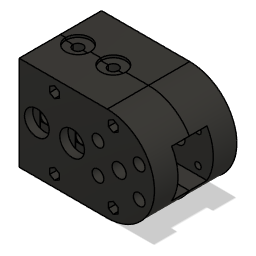
side brace lower mount v4 (Autodesk Fusion 360 design; units mm, degrees)
Autodesk Fusion 360 part; units mm, degrees
sketch "Sketch1" plane through (0, 0, 0) normal (0, 0, 1) x (1, 0, 0)
  line L0 (0, 20.1) -> (0, -20.1)
  line L1 (0, 20.1) -> (-60, 20.1)
  line L2 (-60, 20.1) -> (-60, 40.1)
  line L3 (-60, 40.1) -> (14.9, 40.1)
  circle A0 centre (25, 0) radius 6
  line L4 (0, -20.1) -> (-60, -20.1)
  line L5 (-60, -20.1) -> (-60, -40.1)
  line L6 (-60, -40.1) -> (14.9, -40.1)
  circle A1 centre (25, 0) radius 12.5
  line L7 (0, 0) -> (25, 0) construction
  line L8 (25, 0) -> (55, 0) construction
  arc A2 (14.9, -40.1) -> (14.9, 40.1) centre (14.9, 0) ccw
  dimension "d1" = 40.2
  dimension "d2" = 60
  dimension "d3" = 20
  dimension "d4" = 12
  dimension "d6" = 25
  dimension "d7" = 25
  dimension "d14" = 30
  constraint vertical L0
  constraint midpoint L7.start L0
  constraint perpendicular L0 L1
  constraint perpendicular L1 L2
  constraint perpendicular L2 L3
  constraint perpendicular L2 L4
  constraint perpendicular L1 L5
  constraint perpendicular L5 L6
  constraint equal L2 L5
  constraint collinear L2 L5
  constraint concentric A0 A1
  constraint coincident L7.start origin
  constraint coincident A0.centre A1.centre
  constraint horizontal L7
  constraint parallel L7 L8
  constraint coincident L7 A2.centre
  constraint tangent L3 A2
  constraint coincident L8.end A2
  measures "d1" distance of L0.start L0.end
  measures "d2" distance of L0.start L1.end
  measures "d3" distance of L1.end L2.end
  measures "d4" diameter of A0
  measures "d6" diameter of A1
  measures "d7" distance of L0 A0.centre
  measures "d14" distance of A0.centre L8.end
extrude "Extrude1" add sketch "Sketch1" along normal blind 20 contours L0 L1 L2 L3 L4 L5 L6 A2 | A1 makes body 1
sketch "Sketch3" plane through (0, 0, 0) normal (0, 0, -1) x (-1, 0, 0)
  circle A0 centre (-25, 0) radius 6
  line L0 (0, -20.1) -> (0, 20.1)
  line L1 (0, 20.1) -> (60, 20.1)
  line L2 (60, 20.1) -> (60, 40.1)
  line L3 (60, 40.1) -> (-14.9, 40.1)
  line L4 (-14.9, -40.1) -> (60, -40.1)
  line L5 (60, -40.1) -> (60, -20.1)
  line L6 (60, -20.1) -> (0, -20.1)
  line L7 (60, 20.1) -> (60, -20.1)
  arc A1 (-14.9, 40.1) -> (-14.9, -40.1) centre (-14.9, 0) ccw
  constraint coincident L1.end L2.start
  constraint coincident L5.end L6.start
extrude "Extrude3" add sketch "Sketch3" along normal blind 15 bodies 1
sketch "Sketch4" plane through (0, 0, 20) normal (0, 0, 1) x (1, 0, 0)
  circle A0 centre (25, 0) radius 6
  line L0 (0, 20.1) -> (0, -20.1)
  line L1 (0, -20.1) -> (-60, -20.1)
  line L2 (-60, -20.1) -> (-60, -40.1)
  line L3 (-60, -40.1) -> (14.9, -40.1)
  arc A1 (14.9, -40.1) -> (14.9, 40.1) centre (14.9, 0) ccw
  line L4 (14.9, 40.1) -> (-60, 40.1)
  line L5 (-60, 40.1) -> (-60, 20.1)
  line L6 (-60, 20.1) -> (0, 20.1)
  line L7 (0, 20.1) -> (65, 20.1)
  line L8 (65, 20.1) -> (65, -20.1)
  line L9 (65, -20.1) -> (0, -20.1)
  dimension "d15" = 40
  constraint coincident L0.start L6.end
  constraint perpendicular L0 L7
  constraint perpendicular L1 L8
  constraint coincident L0.end L1.start
  constraint perpendicular L0 L9
  measures "d15" distance of A0.centre L8
extrude "Extrude4" cut sketch "Sketch4" against normal blind 15 contours L0 A1 L7 L9 | A1 L7 L8 L9 bodies 1
sketch "Sketch5" plane through (0, 0, 0) normal (0, 0, 1) x (1, 0, 0)
  line L0 (0, 20.1) -> (-60, 20.1)
  line L1 (-60, 20.1) -> (-60, -20.1)
  line L2 (-60, -20.1) -> (0, -20.1)
  line L3 (0, -20.1) -> (0, 20.1)
  line L4 (-30, 20.1) -> (-30, -20.1) construction
  line L5 (-60, 0) -> (-30, 0) construction
  line L6 (0, 0) -> (-30, 0) construction
  circle A0 centre (-45, 0) radius 10.5
  circle A1 centre (-15, 0) radius 10.5
  circle A2 centre (-45, 0) radius 4.25
  circle A3 centre (-15, 0) radius 4.25
  dimension "d18" = 21
  dimension "d19" = 21
  dimension "d20" = 8.5
  dimension "d21" = 8.5
  constraint midpoint L0 L4.start
  constraint midpoint L2 L4.end
  constraint midpoint L1 L5.start
  constraint midpoint L4 L5.end
  constraint coincident L6.start origin
  constraint midpoint L5 A0.centre
  constraint midpoint L6 A1.centre
  constraint concentric A0 A2
  constraint concentric A1 A3
  measures "d18" diameter of A0
  measures "d19" diameter of A1
  measures "d20" diameter of A2
  measures "d21" diameter of A3
extrude "Extrude5" cut sketch "Sketch5" against normal blind 18 contours A0 | A1 | A2 | A3 bodies 1
extrude "Extrude6" add sketch "Sketch5" against normal blind 8 contours A0 | A1 bodies 1
sketch "Sketch6" plane through (0, 20.1, 0) normal (0, -1, 0) x (1, 0, 0)
  line L0 (-60, 0) -> (0, 0)
  line L1 (0, 0) -> (0, 5)
  line L2 (0, 5) -> (49.5987, 5)
  line L3 (49.5987, 5) -> (49.5987, 20)
  line L4 (49.5987, 20) -> (-60, 20)
  line L5 (-60, 20) -> (-60, 0)
  line L6 (0, 5) -> (0, 20) construction
  line L7 (-30, 0) -> (-30, 20) construction
  line L8 (-30, 20) -> (-60, 20) construction
  line L9 (-30, 20) -> (0, 20) construction
  circle A0 centre (-45, 20) radius 10.5
  circle A1 centre (-15, 20) radius 10.5
  circle A2 centre (-45, 20) radius 4.25
  circle A3 centre (-15, 20) radius 4.25
  dimension "d26" = 21
  dimension "d27" = 21
  dimension "d28" = 8.5
  dimension "d29" = 8.5
  constraint coincident L1.end L2.start
  constraint coincident L4 L6.end
  constraint perpendicular L4 L6
  constraint midpoint L0 L7.start
  constraint coincident L4 L7.end
  constraint perpendicular L4 L7
  constraint coincident L4.end L5.start
  constraint midpoint L8 A0.centre
  constraint midpoint L9 A1.centre
  constraint concentric A0 A2
  constraint concentric A1 A3
  measures "d26" diameter of A0
  measures "d27" diameter of A1
  measures "d28" diameter of A2
  measures "d29" diameter of A3
extrude "Extrude7" cut sketch "Sketch6" along normal blind -20 and the other way blind -88 contours L4 A0 A2 | L4 A2 | L4 A1 A3 | L4 A3 picked at (-53.3618, 19.2672) picked at (-43.8015, 17.5113) picked at (-23.3776, 19.4784) picked at (-15.8675, 18.6813) bodies 1
extrude "Extrude8" add sketch "Sketch6" against normal blind 18 contours L4 A0 A2 | L4 A1 A3 picked at (-53.3618, 19.2672) picked at (-23.3776, 19.4784) bodies 1
extrude "Extrude9" add sketch "Sketch6" along normal blind 18 from surface at 40.2 contours L4 A0 A2 | L4 A1 A3 picked at (-53.3618, 19.2672) picked at (-23.3776, 19.4784) bodies 1
sketch "Sketch7" plane through (0, 0, -15) normal (0, 0, -1) x (-1, 0, 0)
  circle A0 centre (45, 0) radius 10.5
  circle A1 centre (15, 0) radius 10.5
  circle A2 centre (-25, 0) radius 6
  line L0 (60, -40.1) -> (60, 40.1)
  line L1 (60, 40.1) -> (-14.9, 40.1)
  arc A3 (-14.9, 40.1) -> (-14.9, -40.1) centre (-14.9, 0) ccw
  line L2 (-14.9, -40.1) -> (60, -40.1)
  line L3 (-42, 12.9) -> (-7, 12.9) construction
  line L4 (-42, 12.9) -> (-42, -12.9) construction
  line L5 (-42, -12.9) -> (-7, -12.9) construction
  line L6 (-42, 0) -> (-25, 0) construction
  circle A4 centre (-42, -12.9) radius 5
  circle A5 centre (-42, 12.9) radius 5
  circle A6 centre (-7, 12.9) radius 5
  circle A7 centre (-7, -12.9) radius 5
  circle A8 centre (-7, -12.9) radius 2.7
  circle A9 centre (-42, -12.9) radius 2.7
  circle A10 centre (-42, 12.9) radius 2.7
  circle A11 centre (-7, 12.9) radius 2.7
  line L7 (15, 0) -> (45, 0) construction
  line L8 (30, 0) -> (30, 30.1) construction
  circle A12 centre (30, 30.1) radius 5
  circle A13 centre (30, 30.1) radius 2.7
  line L9 (30, 30.1) -> (-20, 30.1) construction
  circle A14 centre (-20, 30.1) radius 5
  circle A15 centre (-20, 30.1) radius 2.7
  circle A16 centre (-20, -30.1) radius 5
  circle A17 centre (-20, -30.1) radius 2.7
  circle A18 centre (30, -30.1) radius 5
  circle A19 centre (30, -30.1) radius 2.7
  dimension "d39" = 35
  dimension "d40" = 18
  dimension "d41" = 25.8
  dimension "d42" = 10
  dimension "d43" = 5.4
  dimension "d44" = 10
  dimension "d45" = 5.4
  dimension "d46" = 10
  dimension "d47" = 50
  dimension "d48" = 10
  dimension "d49" = 5.4
  constraint horizontal L3
  constraint perpendicular L3 L4
  constraint perpendicular L4 L5
  constraint midpoint L4 L6.start
  constraint coincident A2.centre L6.end
  constraint horizontal L6
  constraint equal L3 L5
  constraint coincident L4.end L5.start
  constraint coincident L3.start L4.start
  constraint coincident L3.end A6.centre
  constraint coincident L5.end A7.centre
  constraint equal A6 A7
  constraint equal A5 A6
  constraint equal A4 A5
  constraint concentric A7 A8
  constraint concentric A4 A9
  constraint concentric A5 A10
  constraint concentric A6 A11
  constraint equal A8 A11
  constraint equal A8 A10
  constraint equal A8 A9
  constraint coincident A1.centre L7.start
  constraint coincident A0.centre L7.end
  constraint midpoint L7 L8.start
  constraint perpendicular L7 L8
  constraint coincident L8.end A12.centre
  constraint concentric A12 A13
  constraint perpendicular L8 L9
  constraint coincident L9.end A14.centre
  constraint concentric A14 A15
  constraint symmetric L7 A12 A18
  constraint symmetric L7 A13 A19
  constraint symmetric L7 A14 A16
  constraint symmetric L7 A15 A17
  measures "d39" distance of L3.start L3.end
  measures "d40" horizontal distance of A2.centre L3.end
  measures "d41" distance of L3.start L4.end
  measures "d42" diameter of A7
  measures "d43" diameter of A8
  measures "d44" diameter of A12
  measures "d45" diameter of A13
  measures "d46" distance of L1 L8.end
  measures "d47" distance of L8.end L9.end
  measures "d48" diameter of A14
  measures "d49" diameter of A15
extrude "Extrude10" cut sketch "Sketch7" against normal blind 70 contours A8 | A9 | A10 | A11 | A13 | A15 | A17 | A19 bodies 1
extrude "Extrude12" cut sketch "Sketch7" against normal blind 12 contours A4 | A5 | A6 | A7 bodies 1
mirror "Mirror1" about plane through (0, 0, 20) normal (0, 0, 1) of bodies 1 makes body 2
extrude "Extrude13" cut sketch "Sketch7" against normal blind 15 contours A12 | A14 | A16 | A18 bodies 1
sketch "Sketch8" plane through (0, 0, 55) normal (0, 0, 1) x (1, 0, 0)
  circle A0 centre (7, 12.9) radius 5
  circle A1 centre (7, -12.9) radius 5
  circle A2 centre (42, 12.9) radius 5
  circle A3 centre (42, -12.9) radius 5
  circle A4 centre (-30, -30.1) radius 2.7
  circle A5 centre (-30, 30.1) radius 2.7
  circle A6 centre (20, -30.1) radius 2.7
  circle A7 centre (20, 30.1) radius 2.7
  circle A8 centre (-45, 0) radius 10.5
  circle A9 centre (-15, 0) radius 10.5
  circle A10 centre (25, 0) radius 6
  line L0 (-60, 40.1) -> (-60, -40.1)
  line L1 (-60, -40.1) -> (14.9, -40.1)
  arc A11 (14.9, -40.1) -> (14.9, 40.1) centre (14.9, 0) ccw
  line L2 (14.9, 40.1) -> (-60, 40.1)
  line L3 (-25.9, 32.4671) -> (-30, 34.8343)
  line L4 (-30, 34.8343) -> (-34.1, 32.4671)
  line L5 (-34.1, 32.4671) -> (-34.1, 27.7329)
  line L6 (-34.1, 27.7329) -> (-30, 25.3657)
  line L7 (-30, 25.3657) -> (-25.9, 27.7329)
  line L8 (-25.9, 27.7329) -> (-25.9, 32.4671)
  line L9 (15.9, 27.7329) -> (20, 25.3657)
  line L10 (20, 25.3657) -> (24.1, 27.7329)
  line L11 (24.1, 27.7329) -> (24.1, 32.4671)
  line L12 (24.1, 32.4671) -> (20, 34.8343)
  line L13 (20, 34.8343) -> (15.9, 32.4671)
  line L14 (15.9, 32.4671) -> (15.9, 27.7329)
  line L15 (-25.9, -27.7329) -> (-30, -25.3657)
  line L16 (-30, -25.3657) -> (-34.1, -27.7329)
  line L17 (-34.1, -27.7329) -> (-34.1, -32.4671)
  line L18 (-34.1, -32.4671) -> (-30, -34.8343)
  line L19 (-30, -34.8343) -> (-25.9, -32.4671)
  line L20 (-25.9, -32.4671) -> (-25.9, -27.7329)
  line L21 (24.1, -27.7329) -> (20, -25.3657)
  line L22 (20, -25.3657) -> (15.9, -27.7329)
  line L23 (15.9, -27.7329) -> (15.9, -32.4671)
  line L24 (15.9, -32.4671) -> (20, -34.8343)
  line L25 (20, -34.8343) -> (24.1, -32.4671)
  line L26 (24.1, -32.4671) -> (24.1, -27.7329)
  point P0 (-30, 30.1)
  point P1 (20, 30.1)
  point P2 (-30, -30.1)
  point P3 (20, -30.1)
  dimension "d66" = 8.2
  constraint coincident P0 A5.centre
  constraint coincident P1 A7.centre
  constraint coincident P2 A4.centre
  constraint coincident P3 A6.centre
  constraint equal L8 L14
  constraint equal L14 L23
  constraint equal L20 L23
  constraint vertical L8
  constraint vertical L14
  constraint vertical L23
  constraint vertical L20
  measures "d66" distance of L5 L8
extrude "Extrude14" cut sketch "Sketch8" against normal blind 20 contours A4 | A5 | A7 | L3 L4 L5 L6 L7 L8 | L9 L10 L11 L12 L13 L14 | L15 L16 L17 L18 L19 L20 | L21 L22 L23 L24 L25 L26 bodies 2
copy_body "Body->Comp1" bodies 1 removing the originals makes body 3 in component "side brace lwr mount RH"
copy_body "Body->Comp2" bodies 2 removing the originals makes body 4 in component "side brace lwr mount LH"
sketch "Sketch9" plane through (0, 0, 0) normal (0, 0, -1) x (-1, 0, 0)
  circle A0 centre (-20, 30.1) radius 2.7
  circle A1 centre (-20, 30.1) radius 5
  circle A2 centre (30, 30.1) radius 2.7
  circle A3 centre (30, 30.1) radius 5
  circle A4 centre (30, -30.1) radius 2.7
  circle A5 centre (30, -30.1) radius 5
  circle A6 centre (-20, -30.1) radius 2.7
  circle A7 centre (-20, -30.1) radius 5
  line L0 (-20, -30.1) -> (30, -30.1) construction
  line L1 (-20, 30.1) -> (30, 30.1) construction
  line L2 (5, 30.1) -> (5, -30.1) construction
  line L3 (5, 0) -> (-16, 0) construction
  line L4 (-22.7, 34.3083) -> (-22.7, 25.8917)
  line L5 (-17.3, 34.3083) -> (-17.3, 25.8917)
  line L6 (-17.3, 32.8) -> (-22.7, 32.8)
  line L7 (-22.7, 27.4) -> (-17.3, 27.4)
  line L8 (27.3, 32.8) -> (32.7, 32.8)
  line L9 (32.7, 34.3083) -> (32.7, 25.8917)
  line L10 (32.7, 27.4) -> (27.3, 27.4)
  line L11 (27.3, 34.3083) -> (27.3, 25.8917)
  line L12 (-22.7, -34.3083) -> (-22.7, -25.8917)
  line L13 (-17.3, -32.8) -> (-22.7, -32.8)
  line L14 (-17.3, -34.3083) -> (-17.3, -25.8917)
  line L15 (-22.7, -27.4) -> (-17.3, -27.4)
  line L16 (27.3, -34.3083) -> (27.3, -25.8917)
  line L17 (27.3, -32.8) -> (32.7, -32.8)
  line L18 (32.7, -34.3083) -> (32.7, -25.8917)
  line L19 (32.7, -27.4) -> (27.3, -27.4)
  constraint coincident A6.centre A7.centre
  constraint coincident A4.centre A5.centre
  constraint coincident A0.centre A1.centre
  constraint coincident A2.centre A3.centre
  constraint midpoint L1 L2.start
  constraint midpoint L0 L2.end
  constraint midpoint L2 L3.start
  constraint perpendicular L2 L3
  constraint coincident A1 L4.start
  constraint coincident A1 L4.end
  constraint vertical L4
  constraint coincident A1 L5.start
  constraint coincident A1 L5.end
  constraint perpendicular L1 L5
  constraint coincident L5 L6.start
  constraint coincident L4 L6.end
  constraint perpendicular L4 L6
  constraint coincident L4 L7.start
  constraint coincident L5 L7.end
  constraint perpendicular L5 L7
  constraint tangent A0 L6
  constraint tangent A0 L5
  constraint tangent A0 L7
  constraint tangent A0 L4
  constraint symmetric L2 L4.start L9.start
  constraint symmetric L2 L4.end L9.end
  constraint symmetric L2 L5.start L11.start
  constraint symmetric L2 L5.end L11.end
  constraint symmetric L2 L6.start L8.start
  constraint symmetric L2 L6.end L8.end
  constraint symmetric L2 L7.start L10.start
  constraint symmetric L2 L7.end L10.end
  constraint symmetric L3 L4.start L12.start
  constraint symmetric L3 L4.end L12.end
  constraint symmetric L3 L5.start L14.start
  constraint symmetric L3 L5.end L14.end
  constraint symmetric L3 L6.start L13.start
  constraint symmetric L3 L6.end L13.end
  constraint symmetric L3 L7.start L15.start
  constraint symmetric L3 L7.end L15.end
  constraint symmetric L3 L8.start L17.start
  constraint symmetric L3 L8.end L17.end
  constraint symmetric L3 L9.start L18.start
  constraint symmetric L3 L9.end L18.end
  constraint symmetric L3 L10.start L19.start
  constraint symmetric L3 L10.end L19.end
  constraint symmetric L3 L11.start L16.start
  constraint symmetric L3 L11.end L16.end
extrude "Extrude1'" cut sketch "Sketch9" against normal blind 0.2 contours A0 L5 L7 | A0 L5 L6 | A1 L4 L5 L6 | A0 L4 L6 | A0 L4 L7 | A1 L4 L5 L7 | A2 L9 L10 | A2 L8 L9 | A2 L8 L11 | A3 L8 L9 L11 | A2 L10 L11 | A3 L9 L10 L11 | A4 L17 L18 | A4 L18 L19 | A5 L16 L18 L19 | A4 L16 L19 | A4 L16 L17 | A5 L16 L17 L18 | A6 L13 L14 | A6 L14 L15 | A6 L12 L15 | A7 L12 L14 L15 | A6 L12 L13 | A7 L12 L13 L14 bodies 3 in component "side brace lwr mount RH"
extrude "Extrude2" cut sketch "Sketch9" against normal blind 0.4 contours A0 L5 L7 | A0 L5 L6 | A0 L4 L6 | A0 L4 L7 | A2 L9 L10 | A2 L8 L9 | A2 L8 L11 | A2 L10 L11 | A4 L17 L18 | A4 L18 L19 | A4 L16 L19 | A4 L16 L17 | A6 L13 L14 | A6 L14 L15 | A6 L12 L15 | A6 L12 L13 bodies 3 in component "side brace lwr mount RH"
sketch "Sketch10" plane through (0, 0, -8) normal (0, 0, -1) x (-1, 0, 0)
  circle A0 centre (15, 0) radius 4.25
  circle A1 centre (15, 0) radius 10.5
  circle A2 centre (45, 0) radius 4.25
  circle A3 centre (45, 0) radius 10.5
  line L0 (10.75, 9.6014) -> (10.75, -9.6014)
  line L1 (10.75, -4.25) -> (19.25, -4.25)
  line L2 (19.25, 9.6014) -> (19.25, -9.6014)
  line L3 (19.25, 4.25) -> (10.75, 4.25)
  line L4 (40.75, 9.6014) -> (40.75, -9.6014)
  line L5 (49.25, 9.6014) -> (49.25, -9.6014)
  line L6 (49.25, -4.25) -> (40.75, -4.25)
  line L7 (40.75, 4.25) -> (49.25, 4.25)
  constraint coincident A1 L0.start
  constraint coincident A1 L0.end
  constraint vertical L0
  constraint coincident L0 L1.start
  constraint perpendicular L0 L1
  constraint coincident A1 L2.start
  constraint coincident A1 L2.end
  constraint vertical L2
  constraint coincident L2 L3.start
  constraint coincident L0 L3.end
  constraint perpendicular L0 L3
  constraint coincident L1.end L2
  constraint tangent A0 L2
  constraint tangent A0 L3
  constraint tangent A0 L0
  constraint tangent A0 L1
  constraint coincident A3 L4.start
  constraint coincident A3 L4.end
  constraint vertical L4
  constraint coincident A3 L5.start
  constraint coincident A3 L5.end
  constraint parallel L4 L5
  constraint coincident L5 L6.start
  constraint coincident L4 L6.end
  constraint perpendicular L4 L6
  constraint coincident L4 L7.start
  constraint coincident L5 L7.end
  constraint perpendicular L5 L7
  constraint tangent A2 L7
  constraint tangent A2 L5
  constraint tangent A2 L6
  constraint tangent A2 L4
extrude "Extrude3'" cut sketch "Sketch10" against normal blind 0.2 contours A1 L0 L2 L3 | A1 L0 L1 L2 | A3 L4 L5 L7 | A3 L4 L5 L6 bodies 3 in component "side brace lwr mount RH"
extrude "Extrude4'" cut sketch "Sketch10" against normal blind 0.4 contours A0 L1 L2 | A0 L2 L3 | A0 L0 L3 | A0 L0 L1 | A2 L5 L6 | A2 L5 L7 | A2 L4 L7 | A2 L4 L6 bodies 3 in component "side brace lwr mount RH"
sketch "Sketch11" plane through (0, 0, -3) normal (0, 0, -1) x (-1, 0, 0)
  circle A0 centre (-42, 12.9) radius 2.7
  circle A1 centre (-42, 12.9) radius 5
  circle A2 centre (-7, 12.9) radius 2.7
  circle A3 centre (-7, 12.9) radius 5
  circle A4 centre (-7, -12.9) radius 2.7
  circle A5 centre (-7, -12.9) radius 5
  circle A6 centre (-42, -12.9) radius 2.7
  circle A7 centre (-42, -12.9) radius 5
  line L0 (-42, 12.9) -> (-7, 12.9) construction
  line L1 (-42, -12.9) -> (-7, -12.9) construction
  line L2 (-24.5, 12.9) -> (-24.5, -12.9) construction
  line L3 (-24.5, 0) -> (-36, 0) construction
  line L4 (-44.7, 17.1083) -> (-44.7, 8.6917)
  line L5 (-39.3, 8.6917) -> (-39.3, 17.1083)
  line L6 (-39.3, 15.6) -> (-44.7, 15.6)
  line L7 (-44.7, 10.2) -> (-39.3, 10.2)
  line L8 (-9.7, 15.6) -> (-4.3, 15.6)
  line L9 (-4.3, 17.1083) -> (-4.3, 8.6917)
  line L10 (-9.7, 8.6917) -> (-9.7, 17.1083)
  line L11 (-4.3, 10.2) -> (-9.7, 10.2)
  line L12 (-39.3, -15.6) -> (-44.7, -15.6)
  line L13 (-39.3, -8.6917) -> (-39.3, -17.1083)
  line L14 (-44.7, -10.2) -> (-39.3, -10.2)
  line L15 (-44.7, -17.1083) -> (-44.7, -8.6917)
  line L16 (-4.3, -10.2) -> (-9.7, -10.2)
  line L17 (-9.7, -8.6917) -> (-9.7, -17.1083)
  line L18 (-9.7, -15.6) -> (-4.3, -15.6)
  line L19 (-4.3, -17.1083) -> (-4.3, -8.6917)
  constraint coincident A0.centre A1.centre
  constraint coincident A2.centre A3.centre
  constraint coincident A6.centre A7.centre
  constraint coincident A4.centre A5.centre
  constraint midpoint L0 L2.start
  constraint midpoint L1 L2.end
  constraint midpoint L2 L3.start
  constraint perpendicular L2 L3
  constraint coincident A1 L4.start
  constraint coincident A1 L4.end
  constraint vertical L4
  constraint coincident A1 L5.start
  constraint coincident A1 L5.end
  constraint parallel L4 L5
  constraint coincident L5 L6.start
  constraint coincident L4 L6.end
  constraint perpendicular L4 L6
  constraint coincident L4 L7.start
  constraint coincident L5 L7.end
  constraint perpendicular L5 L7
  constraint tangent A0 L7
  constraint tangent A0 L5
  constraint tangent A0 L6
  constraint tangent A0 L4
  constraint symmetric L2 L4.start L9.start
  constraint symmetric L2 L4.end L9.end
  constraint symmetric L2 L5.start L10.start
  constraint symmetric L2 L5.end L10.end
  constraint symmetric L2 L6.start L8.start
  constraint symmetric L2 L6.end L8.end
  constraint symmetric L2 L7.start L11.start
  constraint symmetric L2 L7.end L11.end
  constraint symmetric L3 L4.start L15.start
  constraint symmetric L3 L4.end L15.end
  constraint symmetric L3 L5.start L13.start
  constraint symmetric L3 L5.end L13.end
  constraint symmetric L3 L6.start L12.start
  constraint symmetric L3 L6.end L12.end
  constraint symmetric L3 L7.start L14.start
  constraint symmetric L3 L7.end L14.end
  constraint symmetric L3 L8.start L18.start
  constraint symmetric L3 L8.end L18.end
  constraint symmetric L3 L9.start L19.start
  constraint symmetric L3 L9.end L19.end
  constraint symmetric L3 L10.start L17.start
  constraint symmetric L3 L10.end L17.end
  constraint symmetric L3 L11.start L16.start
  constraint symmetric L3 L11.end L16.end
extrude "Extrude5'" cut sketch "Sketch11" against normal blind 0.2 contours A1 L4 L5 L6 | A1 L4 L5 L7 | A3 L8 L9 L10 | A3 L9 L10 L11 | A5 L16 L17 L19 | A5 L17 L18 L19 | A7 L13 L14 L15 | A7 L12 L13 L15 bodies 3 in component "side brace lwr mount RH"
extrude "Extrude6'" cut sketch "Sketch11" against normal blind 0.4 contours A0 L5 L7 | A0 L5 L6 | A0 L4 L6 | A0 L4 L7 | A2 L9 L11 | A2 L8 L9 | A2 L8 L10 | A2 L10 L11 | A4 L18 L19 | A4 L16 L19 | A4 L16 L17 | A4 L17 L18 | A6 L12 L13 | A6 L13 L14 | A6 L14 L15 | A6 L12 L15 bodies 3 in component "side brace lwr mount RH"
sketch "Sketch12" plane through (0, 0, 48) normal (0, 0, 1) x (1, 0, 0)
  circle A0 centre (-45, 0) radius 4.25
  circle A1 centre (-45, 0) radius 10.5
  circle A2 centre (-15, 0) radius 4.25
  circle A3 centre (-15, 0) radius 10.5
  line L0 (-49.25, 9.6014) -> (-49.25, -9.6014)
  circle A4 centre (-45, 0) radius 10.5
  line L1 (-40.75, -9.6014) -> (-40.75, 9.6014)
  line L2 (-40.75, 4.25) -> (-49.25, 4.25)
  line L3 (-49.25, -4.25) -> (-40.75, -4.25)
  line L4 (-19.25, 9.6014) -> (-19.25, -9.6014)
  line L5 (-10.75, -9.6014) -> (-10.75, 9.6014)
  line L6 (-10.75, 4.25) -> (-19.25, 4.25)
  line L7 (-19.25, -4.25) -> (-10.75, -4.25)
  constraint coincident A1 L0.start
  constraint vertical L0
  constraint coincident L0.end A4
  constraint coincident A4 L1.start
  constraint coincident A4 L1.end
  constraint vertical L1
  constraint coincident L1 L2.start
  constraint coincident L0 L2.end
  constraint perpendicular L0 L2
  constraint coincident L0 L3.start
  constraint coincident L1 L3.end
  constraint perpendicular L1 L3
  constraint tangent A0 L3
  constraint tangent A0 L1
  constraint tangent A0 L2
  constraint tangent A0 L0
  constraint coincident A3 L4.start
  constraint coincident A3 L4.end
  constraint vertical L4
  constraint coincident A3 L5.start
  constraint coincident A3 L5.end
  constraint parallel L4 L5
  constraint coincident L5 L6.start
  constraint coincident L4 L6.end
  constraint perpendicular L4 L6
  constraint coincident L4 L7.start
  constraint coincident L5 L7.end
  constraint perpendicular L5 L7
  constraint tangent A2 L7
  constraint tangent A2 L5
  constraint tangent A2 L6
  constraint tangent A2 L4
extrude "Extrude1''" cut sketch "Sketch12" against normal blind 0.2 contours A1 L0 A4 L1 L2 | A1 L0 A4 L1 L3 | A3 L4 L5 L6 | A3 L4 L5 L7 bodies 4 in component "side brace lwr mount LH"
extrude "Extrude2'" cut sketch "Sketch12" against normal blind 0.4 contours A0 L1 L3 | A0 L1 L2 | A0 L0 L2 | A0 L0 L3 | A2 L5 L7 | A2 L5 L6 | A2 L4 L6 | A2 L4 L7 bodies 4 in component "side brace lwr mount LH"
sketch "Sketch13" plane through (0, 0, 43) normal (0, 0, 1) x (1, 0, 0)
  circle A0 centre (7, 12.9) radius 2.7
  circle A1 centre (7, 12.9) radius 5
  circle A2 centre (42, 12.9) radius 2.7
  circle A3 centre (42, 12.9) radius 5
  circle A4 centre (42, -12.9) radius 2.7
  circle A5 centre (42, -12.9) radius 5
  circle A6 centre (7, -12.9) radius 2.7
  circle A7 centre (7, -12.9) radius 5
  line L0 (4.3, 17.1083) -> (4.3, 8.6917)
  line L1 (9.7, 17.1083) -> (9.7, 8.6917)
  line L2 (9.7, 10.2) -> (4.3, 10.2)
  line L3 (4.3, 15.6) -> (9.7, 15.6)
  circle A8 centre (25, 0) radius 6
  line L4 (25, 0) -> (35.0938, 0) construction
  line L5 (42, 12.9) -> (7, 12.9) construction
  line L6 (24.5, 12.9) -> (24.5, -2) construction
  line L7 (44.7, 15.6) -> (39.3, 15.6)
  line L8 (44.7, 17.1083) -> (44.7, 8.6917)
  line L9 (39.3, 17.1083) -> (39.3, 8.6917)
  line L10 (39.3, 10.2) -> (44.7, 10.2)
  line L11 (9.7, -10.2) -> (4.3, -10.2)
  line L12 (4.3, -17.1083) -> (4.3, -8.6917)
  line L13 (4.3, -15.6) -> (9.7, -15.6)
  line L14 (9.7, -17.1083) -> (9.7, -8.6917)
  line L15 (44.7, -15.6) -> (39.3, -15.6)
  line L16 (39.3, -17.1083) -> (39.3, -8.6917)
  line L17 (39.3, -10.2) -> (44.7, -10.2)
  line L18 (44.7, -17.1083) -> (44.7, -8.6917)
  constraint coincident A1 L0.start
  constraint coincident A1 L0.end
  constraint vertical L0
  constraint coincident A1 L1.start
  constraint coincident A1 L1.end
  constraint parallel L0 L1
  constraint coincident L1 L2.start
  constraint coincident L0 L2.end
  constraint perpendicular L0 L2
  constraint coincident L0 L3.start
  constraint coincident L1 L3.end
  constraint perpendicular L1 L3
  constraint coincident A8.centre L4.start
  constraint horizontal L4
  constraint coincident A2.centre A3.centre
  constraint coincident A0.centre A1.centre
  constraint midpoint L5 L6.start
  constraint perpendicular L5 L6
  constraint symmetric L0.start L6 L8.start
  constraint symmetric L0.end L6 L8.end
  constraint symmetric L1.start L6 L9.start
  constraint symmetric L1.end L6 L9.end
  constraint symmetric L2.start L6 L10.start
  constraint symmetric L2.end L6 L10.end
  constraint symmetric L3.start L6 L7.start
  constraint symmetric L3.end L6 L7.end
  constraint symmetric L0.start L4 L12.start
  constraint symmetric L0.end L4 L12.end
  constraint symmetric L1.start L4 L14.start
  constraint symmetric L1.end L4 L14.end
  constraint symmetric L2.start L4 L11.start
  constraint symmetric L2.end L4 L11.end
  constraint symmetric L3.start L4 L13.start
  constraint symmetric L3.end L4 L13.end
  constraint symmetric L4 L7.start L15.start
  constraint symmetric L4 L7.end L15.end
  constraint symmetric L4 L8.start L18.start
  constraint symmetric L4 L8.end L18.end
  constraint symmetric L4 L9.start L16.start
  constraint symmetric L4 L9.end L16.end
  constraint symmetric L4 L10.start L17.start
  constraint symmetric L4 L10.end L17.end
  constraint tangent A0 L2
  constraint tangent A0 L1
  constraint tangent A0 L3
  constraint tangent A0 L0
extrude "Extrude3''" cut sketch "Sketch13" against normal blind 0.2 contours A1 L0 L1 L3 | A1 L0 L1 L2 | A3 L7 L8 L9 | A3 L8 L9 L10 | A5 L16 L17 L18 | A5 L15 L16 L18 | A7 L11 L12 L14 | A7 L12 L13 L14 bodies 4 in component "side brace lwr mount LH"
extrude "Extrude4''" cut sketch "Sketch13" against normal blind 0.4 contours A0 L1 L2 | A0 L1 L3 | A0 L0 L3 | A0 L0 L2 | A2 L8 L10 | A2 L7 L8 | A2 L7 L9 | A2 L9 L10 | A4 L15 L18 | A4 L17 L18 | A4 L16 L17 | A4 L15 L16 | A6 L13 L14 | A6 L11 L14 | A6 L11 L12 | A6 L12 L13 bodies 4 in component "side brace lwr mount LH"
sketch "Sketch14" plane through (0, 0, 35) normal (0, 0, 1) x (1, 0, 0)
  circle A0 centre (-30, 30.1) radius 2.7
  line L0 (-25.9, 27.7329) -> (-25.9, 32.4671)
  line L1 (-25.9, 32.4671) -> (-30, 34.8343)
  line L2 (-30, 34.8343) -> (-34.1, 32.4671)
  line L3 (-34.1, 32.4671) -> (-34.1, 27.7329)
  line L4 (-34.1, 27.7329) -> (-30, 25.3657)
  line L5 (-30, 25.3657) -> (-25.9, 27.7329)
  circle A1 centre (20, 30.1) radius 2.7
  line L6 (15.9, 32.4671) -> (15.9, 27.7329)
  line L7 (15.9, 27.7329) -> (20, 25.3657)
  line L8 (20, 25.3657) -> (24.1, 27.7329)
  line L9 (24.1, 27.7329) -> (24.1, 32.4671)
  line L10 (24.1, 32.4671) -> (20, 34.8343)
  line L11 (20, 34.8343) -> (15.9, 32.4671)
  line L12 (24.1, -32.4671) -> (24.1, -27.7329)
  line L13 (24.1, -27.7329) -> (20, -25.3657)
  line L14 (20, -25.3657) -> (15.9, -27.7329)
  line L15 (15.9, -27.7329) -> (15.9, -32.4671)
  line L16 (15.9, -32.4671) -> (20, -34.8343)
  line L17 (20, -34.8343) -> (24.1, -32.4671)
  circle A2 centre (20, -30.1) radius 2.7
  circle A3 centre (-30, -30.1) radius 2.7
  line L18 (-25.9, -32.4671) -> (-25.9, -27.7329)
  line L19 (-25.9, -27.7329) -> (-30, -25.3657)
  line L20 (-30, -25.3657) -> (-34.1, -27.7329)
  line L21 (-34.1, -27.7329) -> (-34.1, -32.4671)
  line L22 (-34.1, -32.4671) -> (-30, -34.8343)
  line L23 (-30, -34.8343) -> (-25.9, -32.4671)
  line L24 (0, 0) -> (-31, 0) construction
  line L25 (-30, 30.1) -> (20, 30.1) construction
  line L26 (-5, 30.1) -> (-5, 18) construction
  line L27 (-32.7, 33.2754) -> (-32.7, 26.9246)
  line L28 (-27.3, 33.2754) -> (-27.3, 26.9246)
  line L29 (-27.3, 32.8) -> (-32.7, 32.8)
  line L30 (-32.7, 27.4) -> (-27.3, 27.4)
  line L31 (17.3, 32.8) -> (22.7, 32.8)
  line L32 (22.7, 33.2754) -> (22.7, 26.9246)
  line L33 (17.3, 33.2754) -> (17.3, 26.9246)
  line L34 (22.7, 27.4) -> (17.3, 27.4)
  line L35 (-27.3, -32.8) -> (-32.7, -32.8)
  line L36 (-32.7, -33.2754) -> (-32.7, -26.9246)
  line L37 (-27.3, -33.2754) -> (-27.3, -26.9246)
  line L38 (-32.7, -27.4) -> (-27.3, -27.4)
  line L39 (22.7, -27.4) -> (17.3, -27.4)
  line L40 (22.7, -33.2754) -> (22.7, -26.9246)
  line L41 (17.3, -32.8) -> (22.7, -32.8)
  line L42 (17.3, -33.2754) -> (17.3, -26.9246)
  constraint coincident L24.start origin
  constraint horizontal L24
  constraint coincident A0.centre L25.start
  constraint coincident A1.centre L25.end
  constraint midpoint L25 L26.start
  constraint perpendicular L25 L26
  constraint coincident L2 L27.start
  constraint coincident L4 L27.end
  constraint vertical L27
  constraint coincident L1 L28.start
  constraint coincident L5 L28.end
  constraint parallel L27 L28
  constraint coincident L28 L29.start
  constraint coincident L27 L29.end
  constraint perpendicular L27 L29
  constraint coincident L27 L30.start
  constraint coincident L28 L30.end
  constraint perpendicular L28 L30
  constraint tangent A0 L30
  constraint tangent A0 L28
  constraint tangent A0 L29
  constraint tangent A0 L27
  constraint symmetric L26 L27.start L32.start
  constraint symmetric L26 L27.end L32.end
  constraint symmetric L26 L28.start L33.start
  constraint symmetric L26 L28.end L33.end
  constraint symmetric L26 L29.start L31.start
  constraint symmetric L26 L29.end L31.end
  constraint symmetric L26 L30.start L34.start
  constraint symmetric L26 L30.end L34.end
  constraint symmetric L24 L27.start L36.start
  constraint symmetric L24 L27.end L36.end
  constraint symmetric L24 L28.start L37.start
  constraint symmetric L24 L28.end L37.end
  constraint symmetric L24 L29.start L35.start
  constraint symmetric L24 L29.end L35.end
  constraint symmetric L24 L30.start L38.start
  constraint symmetric L24 L30.end L38.end
  constraint symmetric L24 L31.start L41.start
  constraint symmetric L24 L31.end L41.end
  constraint symmetric L24 L32.start L40.start
  constraint symmetric L24 L32.end L40.end
  constraint symmetric L24 L33.start L42.start
  constraint symmetric L24 L33.end L42.end
  constraint symmetric L24 L34.start L39.start
  constraint symmetric L24 L34.end L39.end
extrude "Extrude5''" cut sketch "Sketch14" against normal blind 0.2 contours L1 L2 L27 L28 L29 | L4 L5 L27 L28 L30 | L10 L11 L31 L32 L33 | L7 L8 L32 L33 L34 | L16 L17 L40 L41 L42 | L13 L14 L39 L40 L42 | L19 L20 L36 L37 L38 | L22 L23 L35 L36 L37 bodies 4 in component "side brace lwr mount LH"
extrude "Extrude6''" cut sketch "Sketch14" against normal blind 0.4 contours A0 L28 L30 | A0 L28 L29 | A0 L27 L29 | A0 L27 L30 | A1 L32 L34 | A1 L31 L32 | A1 L31 L33 | A1 L33 L34 | A2 L40 L41 | A2 L39 L40 | A2 L41 L42 | A2 L39 L42 | A3 L35 L37 | A3 L37 L38 | A3 L36 L38 | A3 L35 L36 bodies 4 in component "side brace lwr mount LH"
component "side brace lwr mount RH" placed x (1, 0, 0) y (0, 1, 0) z (0, 0, 1) at (0, 0, 0)
component "side brace lwr mount LH" placed x (1, 0, 0) y (0, 1, 0) z (0, 0, 1) at (0, 0, 0)
equation "d45 = d49"
named bodies: "side brace lwr mount RH", "side brace lwr mount LH"
